Autodesk Inventor part; units mm, degrees
(part 4 of 5)
sketch "Sketch12" plane through (0, 0, 3) normal (0, 0, 1) x (1, 0, 0)
  line L0 (-25.3933, -129) -> (-25.3933, -146.5) projected
  line L1 (-25.3933, -146.5) -> (23.6067, -146.5) projected
  line L2 (23.6067, -146.5) -> (23.6067, -129) projected
  line L3 (23.6067, -129) -> (98, -129) projected
  line L4 (98, -129) -> (98, 184.5) projected
  line L5 (98, 184.5) -> (80.4, 184.5) projected
  line L6 (80.4, 184.5) -> (80.4, 215) projected
  line L7 (80.4, 215) -> (-78, 215) projected
  line L8 (-78, 215) -> (-78, 46.0635) projected
  line L9 (-78, 46.0635) -> (-75, 46.0635) projected
  line L10 (-75, 46.0635) -> (-75, 40.8932) projected
  line L11 (-75, 40.8932) -> (-78, 40.8932) projected
  line L12 (-78, 40.8932) -> (-78, 30.6062) projected
  line L13 (-78, 30.6062) -> (-75, 30.6062) projected
  line L14 (-75, 30.6062) -> (-75, 20.5478) projected
  line L15 (-75, 20.5478) -> (-78, 20.5478) projected
  line L16 (-78, 20.5478) -> (-78, 10.2608) projected
  line L17 (-78, 10.2608) -> (-75, 10.2608) projected
  line L18 (-75, 10.2608) -> (-75, -0.1068) projected
  line L19 (-75, -0.1068) -> (-78, -0.1068) projected
  line L20 (-78, -0.1068) -> (-78, -10.3938) projected
  line L21 (-78, -10.3938) -> (-75, -10.3938) projected
  line L22 (-75, -10.3938) -> (-75, -20.4522) projected
  line L23 (-75, -20.4522) -> (-78, -20.4522) projected
  line L24 (-78, -20.4522) -> (-78, -30.7392) projected
  line L25 (-78, -30.7392) -> (-75, -30.7392) projected
  line L26 (-75, -30.7392) -> (-75, -41.1068) projected
  line L27 (-75, -41.1068) -> (-78, -41.1068) projected
  line L28 (-78, -41.1068) -> (-78, -51.3938) projected
  line L29 (-78, -51.3938) -> (-75, -51.3938) projected
  line L30 (-75, -51.3938) -> (-75, -61.4522) projected
  line L31 (-75, -61.4522) -> (-78, -61.4522) projected
  line L32 (-78, -61.4522) -> (-78, -71.7392) projected
  line L33 (-78, -71.7392) -> (-75, -71.7392) projected
  line L34 (-75, -71.7392) -> (-75, -82.1068) projected
  line L35 (-75, -82.1068) -> (-78, -82.1068) projected
  line L36 (-78, -82.1068) -> (-78, -92.3938) projected
  line L37 (-78, -92.3938) -> (-75, -92.3938) projected
  line L38 (-75, -92.3938) -> (-75, -102.4522) projected
  line L39 (-75, -102.4522) -> (-78, -102.4522) projected
  line L40 (-78, -102.4522) -> (-78, -112.7392) projected
  line L41 (-78, -112.7392) -> (-75, -112.7392) projected
  line L42 (-75, -112.7392) -> (-75, -129) projected
  line L43 (-75, -129) -> (-25.3933, -129) projected
  circle A0 centre (88, 174.5) radius 2.25 projected
  circle A1 centre (88, 131.8987) radius 2.25 projected
  circle A2 centre (88, 58.3987) radius 2.25 projected
  circle A3 centre (88, -117.6237) radius 2.25 projected
  circle A4 centre (-17.8933, -140) radius 2.25 projected
  circle A5 centre (16.1067, -140) radius 2.25 projected
  line L44 (-58.9404, 10.4643) -> (-58.9404, 20.3443) projected
  arc A6 (-55.9404, 23.3443) -> (-58.9404, 20.3443) centre (-55.9404, 20.3443) ccw projected
  line L45 (-55.9404, 23.3443) -> (31.7396, 23.3443) projected
  arc A7 (34.7396, 20.3443) -> (31.7396, 23.3443) centre (31.7396, 20.3443) ccw projected
  line L46 (34.7396, 20.3443) -> (34.7396, 10.4643) projected
  arc A8 (31.7396, 7.4643) -> (34.7396, 10.4643) centre (31.7396, 10.4643) ccw projected
  line L47 (31.7396, 7.4643) -> (-55.9404, 7.4643) projected
  arc A9 (-58.9404, 10.4643) -> (-55.9404, 7.4643) centre (-55.9404, 10.4643) ccw projected
  line L48 (-58.9404, 30.8097) -> (-58.9404, 40.6897) projected
  arc A10 (-55.9404, 43.6897) -> (-58.9404, 40.6897) centre (-55.9404, 40.6897) ccw projected
  line L49 (-55.9404, 43.6897) -> (31.7396, 43.6897) projected
  arc A11 (34.7396, 40.6897) -> (31.7396, 43.6897) centre (31.7396, 40.6897) ccw projected
  line L50 (34.7396, 40.6897) -> (34.7396, 30.8097) projected
  arc A12 (31.7396, 27.8097) -> (34.7396, 30.8097) centre (31.7396, 30.8097) ccw projected
  line L51 (31.7396, 27.8097) -> (-55.9404, 27.8097) projected
  arc A13 (-58.9404, 30.8097) -> (-55.9404, 27.8097) centre (-55.9404, 30.8097) ccw projected
  arc A14 (-55.9404, 2.9989) -> (-58.9404, -0.0011) centre (-55.9404, -0.0011) ccw projected
  line L52 (-55.9404, 2.9989) -> (31.7396, 2.9989) projected
  arc A15 (34.7396, -0.0011) -> (31.7396, 2.9989) centre (31.7396, -0.0011) ccw projected
  line L53 (34.7396, -0.0011) -> (34.7396, -9.8811) projected
  arc A16 (31.7396, -12.8811) -> (34.7396, -9.8811) centre (31.7396, -9.8811) ccw projected
  line L54 (31.7396, -12.8811) -> (-55.9404, -12.8811) projected
  arc A17 (-58.9404, -9.8811) -> (-55.9404, -12.8811) centre (-55.9404, -9.8811) ccw projected
  line L55 (-58.9404, -9.8811) -> (-58.9404, -0.0011) projected
  arc A18 (-55.9404, -37.6919) -> (-58.9404, -40.6919) centre (-55.9404, -40.6919) ccw projected
  line L56 (-55.9404, -37.6919) -> (31.7396, -37.6919) projected
  arc A19 (34.7396, -40.6919) -> (31.7396, -37.6919) centre (31.7396, -40.6919) ccw projected
  line L57 (34.7396, -40.6919) -> (34.7396, -50.5719) projected
  arc A20 (31.7396, -53.5719) -> (34.7396, -50.5719) centre (31.7396, -50.5719) ccw projected
  line L58 (31.7396, -53.5719) -> (-55.9404, -53.5719) projected
  arc A21 (-58.9404, -50.5719) -> (-55.9404, -53.5719) centre (-55.9404, -50.5719) ccw projected
  line L59 (-58.9404, -50.5719) -> (-58.9404, -40.6919) projected
  line L60 (-55.9404, -58.0373) -> (31.7396, -58.0373) projected
  arc A22 (34.7396, -61.0373) -> (31.7396, -58.0373) centre (31.7396, -61.0373) ccw projected
  line L61 (34.7396, -61.0373) -> (34.7396, -70.9173) projected
  arc A23 (31.7396, -73.9173) -> (34.7396, -70.9173) centre (31.7396, -70.9173) ccw projected
  line L62 (31.7396, -73.9173) -> (-55.9404, -73.9173) projected
  arc A24 (-58.9404, -70.9173) -> (-55.9404, -73.9173) centre (-55.9404, -70.9173) ccw projected
  line L63 (-58.9404, -70.9173) -> (-58.9404, -61.0373) projected
  arc A25 (-55.9404, -58.0373) -> (-58.9404, -61.0373) centre (-55.9404, -61.0373) ccw projected
  line L64 (31.7396, -33.2265) -> (-55.9404, -33.2265) projected
  arc A26 (-58.9404, -30.2265) -> (-55.9404, -33.2265) centre (-55.9404, -30.2265) ccw projected
  line L65 (-58.9404, -30.2265) -> (-58.9404, -20.3465) projected
  arc A27 (-55.9404, -17.3465) -> (-58.9404, -20.3465) centre (-55.9404, -20.3465) ccw projected
  line L66 (-55.9404, -17.3465) -> (31.7396, -17.3465) projected
  arc A28 (34.7396, -20.3465) -> (31.7396, -17.3465) centre (31.7396, -20.3465) ccw projected
  line L67 (34.7396, -20.3465) -> (34.7396, -30.2265) projected
  arc A29 (31.7396, -33.2265) -> (34.7396, -30.2265) centre (31.7396, -30.2265) ccw projected
  arc A30 (34.7396, -81.3827) -> (31.7396, -78.3827) centre (31.7396, -81.3827) ccw projected
  line L68 (34.7396, -81.3827) -> (34.7396, -91.2627) projected
  arc A31 (31.7396, -94.2627) -> (34.7396, -91.2627) centre (31.7396, -91.2627) ccw projected
  line L69 (31.7396, -94.2627) -> (-55.9404, -94.2627) projected
  arc A32 (-58.9404, -91.2627) -> (-55.9404, -94.2627) centre (-55.9404, -91.2627) ccw projected
  line L70 (-58.9404, -91.2627) -> (-58.9404, -81.3827) projected
  arc A33 (-55.9404, -78.3827) -> (-58.9404, -81.3827) centre (-55.9404, -81.3827) ccw projected
  line L71 (-55.9404, -78.3827) -> (31.7396, -78.3827) projected
  arc A34 (31.7396, -114.6081) -> (34.7396, -111.6081) centre (31.7396, -111.6081) ccw projected
  line L72 (31.7396, -114.6081) -> (-55.9404, -114.6081) projected
  arc A35 (-58.9404, -111.6081) -> (-55.9404, -114.6081) centre (-55.9404, -111.6081) ccw projected
  line L73 (-58.9404, -111.6081) -> (-58.9404, -101.7281) projected
  arc A36 (-55.9404, -98.7281) -> (-58.9404, -101.7281) centre (-55.9404, -101.7281) ccw projected
  line L74 (-55.9404, -98.7281) -> (31.7396, -98.7281) projected
  arc A37 (34.7396, -101.7281) -> (31.7396, -98.7281) centre (31.7396, -101.7281) ccw projected
  line L75 (34.7396, -101.7281) -> (34.7396, -111.6081) projected
  line L76 (-69.3194, 50.0635) -> (-69.3194, 207.0635) projected
  arc A38 (-68.3194, 208.0635) -> (-69.3194, 207.0635) centre (-68.3194, 207.0635) ccw projected
  line L77 (-68.3194, 208.0635) -> (-25.6194, 208.0635) projected
  arc A39 (-24.6194, 207.0635) -> (-25.6194, 208.0635) centre (-25.6194, 207.0635) ccw projected
  line L78 (-24.6194, 207.0635) -> (-24.6194, 50.0635) projected
  arc A40 (-25.6194, 49.0635) -> (-24.6194, 50.0635) centre (-25.6194, 50.0635) ccw projected
  line L79 (-25.6194, 49.0635) -> (-68.3194, 49.0635) projected
  arc A41 (-69.3194, 50.0635) -> (-68.3194, 49.0635) centre (-68.3194, 50.0635) ccw projected
  line L80 (64, 48.3987) -> (64, -109.7094) projected
  arc A42 (63.7071, -110.4166) -> (64, -109.7094) centre (63, -109.7094) ccw projected
  line L81 (63.7071, -110.4166) -> (59.2929, -114.8308) projected
  arc A43 (58.5858, -115.1237) -> (59.2929, -114.8308) centre (58.5858, -114.1237) ccw projected
  line L82 (58.5858, -115.1237) -> (43.2196, -115.1237) projected
  arc A44 (42.2196, -114.1237) -> (43.2196, -115.1237) centre (43.2196, -114.1237) ccw projected
  line L83 (42.2196, -114.1237) -> (42.2196, -104.6674) projected
  arc A45 (42.2196, -104.6674) -> (40.773, -102.7455) centre (40.2196, -104.6674) ccw projected
  arc A46 (39.7673, -102.1811) -> (40.773, -102.7455) centre (41.4696, -100.3262) ccw projected
  arc A47 (39.1196, -100.7076) -> (39.7673, -102.1811) centre (41.1196, -100.7076) ccw projected
  line L84 (39.1196, -100.7076) -> (39.1196, -95.7515) projected
  arc A48 (39.7673, -94.2779) -> (39.1196, -95.7515) centre (41.1196, -95.7515) ccw projected
  arc A49 (39.937, -94.1354) -> (39.7673, -94.2779) centre (41.4696, -96.1328) ccw projected
  arc A50 (39.937, -94.1354) -> (40.7196, -92.5486) centre (38.7196, -92.5486) ccw projected
  line L85 (40.7196, -92.5486) -> (40.7196, -83.4104) projected
  arc A51 (40.7196, -83.4104) -> (39.937, -81.8236) centre (38.7196, -83.4104) ccw projected
  arc A52 (39.7673, -81.6811) -> (39.937, -81.8236) centre (41.4696, -79.8262) ccw projected
  arc A53 (39.1196, -80.2076) -> (39.7673, -81.6811) centre (41.1196, -80.2076) ccw projected
  line L86 (39.1196, -80.2076) -> (39.1196, -75.2515) projected
  arc A54 (39.7673, -73.7779) -> (39.1196, -75.2515) centre (41.1196, -75.2515) ccw projected
  arc A55 (39.937, -73.6354) -> (39.7673, -73.7779) centre (41.4696, -75.6328) ccw projected
  arc A56 (39.937, -73.6354) -> (40.7196, -72.0486) centre (38.7196, -72.0486) ccw projected
  line L87 (40.7196, -72.0486) -> (40.7196, -62.9104) projected
  arc A57 (40.7196, -62.9104) -> (39.937, -61.3236) centre (38.7196, -62.9104) ccw projected
  arc A58 (39.7673, -61.1811) -> (39.937, -61.3236) centre (41.4696, -59.3262) ccw projected
  arc A59 (39.1196, -59.7076) -> (39.7673, -61.1811) centre (41.1196, -59.7076) ccw projected
  line L88 (39.1196, -59.7076) -> (39.1196, -54.7515) projected
  arc A60 (39.7673, -53.2779) -> (39.1196, -54.7515) centre (41.1196, -54.7515) ccw projected
  arc A61 (39.937, -53.1354) -> (39.7673, -53.2779) centre (41.4696, -55.1328) ccw projected
  arc A62 (39.937, -53.1354) -> (40.7196, -51.5486) centre (38.7196, -51.5486) ccw projected
  line L89 (40.7196, -51.5486) -> (40.7196, -42.4104) projected
  arc A63 (40.7196, -42.4104) -> (39.937, -40.8236) centre (38.7196, -42.4104) ccw projected
  arc A64 (39.7673, -40.6811) -> (39.937, -40.8236) centre (41.4696, -38.8262) ccw projected
  arc A65 (39.1196, -39.2076) -> (39.7673, -40.6811) centre (41.1196, -39.2076) ccw projected
  line L90 (39.1196, -39.2076) -> (39.1196, -34.2515) projected
  arc A66 (39.7673, -32.7779) -> (39.1196, -34.2515) centre (41.1196, -34.2515) ccw projected
  arc A67 (39.937, -32.6354) -> (39.7673, -32.7779) centre (41.4696, -34.6328) ccw projected
  arc A68 (39.937, -32.6354) -> (40.7196, -31.0486) centre (38.7196, -31.0486) ccw projected
  line L91 (40.7196, -31.0486) -> (40.7196, -21.9104) projected
  arc A69 (40.7196, -21.9104) -> (39.937, -20.3236) centre (38.7196, -21.9104) ccw projected
  arc A70 (39.7673, -20.1811) -> (39.937, -20.3236) centre (41.4696, -18.3262) ccw projected
  arc A71 (39.1196, -18.7076) -> (39.7673, -20.1811) centre (41.1196, -18.7076) ccw projected
  line L92 (39.1196, -18.7076) -> (39.1196, -13.7515) projected
  arc A72 (39.7673, -12.2779) -> (39.1196, -13.7515) centre (41.1196, -13.7515) ccw projected
  arc A73 (39.937, -12.1354) -> (39.7673, -12.2779) centre (41.4696, -14.1328) ccw projected
  arc A74 (39.937, -12.1354) -> (40.7196, -10.5486) centre (38.7196, -10.5486) ccw projected
  line L93 (40.7196, -10.5486) -> (40.7196, -1.4104) projected
  arc A75 (40.7196, -1.4104) -> (39.937, 0.1764) centre (38.7196, -1.4104) ccw projected
  arc A76 (39.7673, 0.3189) -> (39.937, 0.1764) centre (41.4696, 2.1738) ccw projected
  arc A77 (39.1196, 1.7924) -> (39.7673, 0.3189) centre (41.1196, 1.7924) ccw projected
  line L94 (39.1196, 1.7924) -> (39.1196, 6.7485) projected
  arc A78 (39.7673, 8.2221) -> (39.1196, 6.7485) centre (41.1196, 6.7485) ccw projected
  arc A79 (39.937, 8.3646) -> (39.7673, 8.2221) centre (41.4696, 6.3672) ccw projected
  arc A80 (39.937, 8.3646) -> (40.7196, 9.9514) centre (38.7196, 9.9514) ccw projected
  line L95 (40.7196, 9.9514) -> (40.7196, 19.0896) projected
  arc A81 (40.7196, 19.0896) -> (39.937, 20.6764) centre (38.7196, 19.0896) ccw projected
  arc A82 (39.7673, 20.8189) -> (39.937, 20.6764) centre (41.4696, 22.6738) ccw projected
  arc A83 (39.1196, 22.2924) -> (39.7673, 20.8189) centre (41.1196, 22.2924) ccw projected
  line L96 (39.1196, 22.2924) -> (39.1196, 27.2485) projected
  arc A84 (39.7673, 28.7221) -> (39.1196, 27.2485) centre (41.1196, 27.2485) ccw projected
  arc A85 (39.937, 28.8646) -> (39.7673, 28.7221) centre (41.4696, 26.8672) ccw projected
  arc A86 (39.937, 28.8646) -> (40.7196, 30.4514) centre (38.7196, 30.4514) ccw projected
  line L97 (40.7196, 30.4514) -> (40.7196, 39.5896) projected
  arc A87 (40.7196, 39.5896) -> (39.937, 41.1764) centre (38.7196, 39.5896) ccw projected
  arc A88 (39.7673, 41.3189) -> (39.937, 41.1764) centre (41.4696, 43.1738) ccw projected
  arc A89 (39.1196, 42.7924) -> (39.7673, 41.3189) centre (41.1196, 42.7924) ccw projected
  line L98 (39.1196, 42.7924) -> (39.1196, 47.7485) projected
  arc A90 (39.7673, 49.2221) -> (39.1196, 47.7485) centre (41.1196, 47.7485) ccw projected
  arc A91 (43.3362, 49.0566) -> (39.7673, 49.2221) centre (41.4696, 47.3672) ccw projected
  arc A92 (43.3362, 49.0566) -> (44.819, 48.3987) centre (44.819, 50.3987) ccw projected
  line L99 (44.819, 48.3987) -> (64, 48.3987) projected
  line L100 (17.2903, 185.473) -> (38.4903, 185.473)
  line L101 (41.4903, 188.473) -> (41.4903, 201.673)
  line L102 (38.4903, 204.673) -> (17.2903, 204.673)
  line L103 (14.2903, 201.673) -> (14.2903, 188.473)
  arc A93 (38.4903, 185.473) -> (41.4903, 188.473) centre (38.4903, 188.473) ccw
  arc A94 (41.4903, 201.673) -> (38.4903, 204.673) centre (38.4903, 201.673) ccw
  arc A95 (17.2903, 204.673) -> (14.2903, 201.673) centre (17.2903, 201.673) ccw
  arc A96 (14.2903, 188.473) -> (17.2903, 185.473) centre (17.2903, 188.473) ccw
  circle A97 centre (47.8903, 195.073) radius 1.75
  circle A98 centre (7.8903, 195.073) radius 1.75
  line L104 (15.5287, 72.6659) -> (40.2515, 72.6659)
  line L105 (40.2515, 150.2659) -> (15.5287, 150.2659)
  line L106 (-8.1099, 127.2849) -> (-8.1099, 95.6469)
  arc A99 (-8.1099, 95.6469) -> (-2.1613, 81.4146) centre (11.8901, 95.6469) ccw
  arc A100 (4.5403, 75.9549) -> (15.5287, 72.6659) centre (15.5287, 92.6659) ccw
  arc A101 (-2.1615, 81.4137) -> (4.5403, 75.9549) centre (27.8907, 111.4659) ccw
  line L107 (27.8901, 106.1082) -> (27.8901, 119.1725)
  line L108 (22.3518, 111.4659) -> (33.8609, 111.4659)
  arc A102 (-2.1613, 141.5172) -> (-8.1099, 127.2849) centre (11.8901, 127.2849) ccw
  arc A103 (15.5287, 150.2659) -> (4.5403, 146.9769) centre (15.5287, 130.2659) ccw
  arc A104 (4.5403, 146.9769) -> (-2.1615, 141.5181) centre (27.8907, 111.4659) ccw
  line L109 (63.8901, 95.6469) -> (63.8901, 127.2849)
  arc A105 (4.5403, 146.9769) -> (-2.1615, 141.5181) centre (27.8907, 111.4659) ccw
  circle A106 centre (-7.8093, 75.7659) radius 1.2
  circle A107 centre (63.5895, 75.7659) radius 1.2
  circle A108 centre (-7.8093, 147.1659) radius 1.2
  circle A109 centre (63.5895, 147.1659) radius 1.2
  circle A110 centre (88, -117.6237) radius 2.25 projected
  circle A111 centre (88, 58.3987) radius 2.25 projected
  circle A112 centre (88, 131.8987) radius 2.25 projected
  circle A113 centre (88, 174.5) radius 2.25 projected
  line L110 (64, -109.7094) -> (64, 48.3987) projected
  line L111 (64, 48.3987) -> (44.819, 48.3987) projected
  arc A114 (43.3362, 49.0566) -> (44.819, 48.3987) centre (44.819, 50.3987) ccw projected
  arc A115 (43.3362, 49.0566) -> (39.7673, 49.2221) centre (41.4696, 47.3672) ccw projected
  arc A116 (39.7673, 49.2221) -> (39.1196, 47.7485) centre (41.1196, 47.7485) ccw projected
  line L112 (39.1196, 47.7485) -> (39.1196, 42.7924) projected
  arc A117 (39.1196, 42.7924) -> (39.7673, 41.3189) centre (41.1196, 42.7924) ccw projected
  arc A118 (39.7673, 41.3189) -> (39.937, 41.1764) centre (41.4696, 43.1738) ccw projected
  arc A119 (40.7196, 39.5896) -> (39.937, 41.1764) centre (38.7196, 39.5896) ccw projected
  line L113 (40.7196, 39.5896) -> (40.7196, 30.4514) projected
  arc A120 (39.937, 28.8646) -> (40.7196, 30.4514) centre (38.7196, 30.4514) ccw projected
  arc A121 (39.937, 28.8646) -> (39.7673, 28.7221) centre (41.4696, 26.8672) ccw projected
  arc A122 (39.7673, 28.7221) -> (39.1196, 27.2485) centre (41.1196, 27.2485) ccw projected
  line L114 (39.1196, 27.2485) -> (39.1196, 22.2924) projected
  arc A123 (39.1196, 22.2924) -> (39.7673, 20.8189) centre (41.1196, 22.2924) ccw projected
  arc A124 (39.7673, 20.8189) -> (39.937, 20.6764) centre (41.4696, 22.6738) ccw projected
  arc A125 (40.7196, 19.0896) -> (39.937, 20.6764) centre (38.7196, 19.0896) ccw projected
  line L115 (40.7196, 19.0896) -> (40.7196, 9.9514) projected
  arc A126 (39.937, 8.3646) -> (40.7196, 9.9514) centre (38.7196, 9.9514) ccw projected
  arc A127 (39.937, 8.3646) -> (39.7673, 8.2221) centre (41.4696, 6.3672) ccw projected
  arc A128 (39.7673, 8.2221) -> (39.1196, 6.7485) centre (41.1196, 6.7485) ccw projected
  line L116 (39.1196, 6.7485) -> (39.1196, 1.7924) projected
  arc A129 (39.1196, 1.7924) -> (39.7673, 0.3189) centre (41.1196, 1.7924) ccw projected
  arc A130 (39.7673, 0.3189) -> (39.937, 0.1764) centre (41.4696, 2.1738) ccw projected
  arc A131 (40.7196, -1.4104) -> (39.937, 0.1764) centre (38.7196, -1.4104) ccw projected
  line L117 (40.7196, -1.4104) -> (40.7196, -10.5486) projected
  arc A132 (39.937, -12.1354) -> (40.7196, -10.5486) centre (38.7196, -10.5486) ccw projected
  arc A133 (39.937, -12.1354) -> (39.7673, -12.2779) centre (41.4696, -14.1328) ccw projected
  arc A134 (39.7673, -12.2779) -> (39.1196, -13.7515) centre (41.1196, -13.7515) ccw projected
  line L118 (39.1196, -13.7515) -> (39.1196, -18.7076) projected
  arc A135 (39.1196, -18.7076) -> (39.7673, -20.1811) centre (41.1196, -18.7076) ccw projected
  arc A136 (39.7673, -20.1811) -> (39.937, -20.3236) centre (41.4696, -18.3262) ccw projected
  arc A137 (40.7196, -21.9104) -> (39.937, -20.3236) centre (38.7196, -21.9104) ccw projected
  line L119 (40.7196, -21.9104) -> (40.7196, -31.0486) projected
  arc A138 (39.937, -32.6354) -> (40.7196, -31.0486) centre (38.7196, -31.0486) ccw projected
  arc A139 (39.937, -32.6354) -> (39.7673, -32.7779) centre (41.4696, -34.6328) ccw projected
  arc A140 (39.7673, -32.7779) -> (39.1196, -34.2515) centre (41.1196, -34.2515) ccw projected
  line L120 (39.1196, -34.2515) -> (39.1196, -39.2076) projected
  arc A141 (39.1196, -39.2076) -> (39.7673, -40.6811) centre (41.1196, -39.2076) ccw projected
  arc A142 (39.7673, -40.6811) -> (39.937, -40.8236) centre (41.4696, -38.8262) ccw projected
  arc A143 (40.7196, -42.4104) -> (39.937, -40.8236) centre (38.7196, -42.4104) ccw projected
  line L121 (40.7196, -42.4104) -> (40.7196, -51.5486) projected
  arc A144 (39.937, -53.1354) -> (40.7196, -51.5486) centre (38.7196, -51.5486) ccw projected
  arc A145 (39.937, -53.1354) -> (39.7673, -53.2779) centre (41.4696, -55.1328) ccw projected
  arc A146 (39.7673, -53.2779) -> (39.1196, -54.7515) centre (41.1196, -54.7515) ccw projected
  line L122 (39.1196, -54.7515) -> (39.1196, -59.7076) projected
  arc A147 (39.1196, -59.7076) -> (39.7673, -61.1811) centre (41.1196, -59.7076) ccw projected
  arc A148 (39.7673, -61.1811) -> (39.937, -61.3236) centre (41.4696, -59.3262) ccw projected
  arc A149 (40.7196, -62.9104) -> (39.937, -61.3236) centre (38.7196, -62.9104) ccw projected
  line L123 (40.7196, -62.9104) -> (40.7196, -72.0486) projected
  arc A150 (39.937, -73.6354) -> (40.7196, -72.0486) centre (38.7196, -72.0486) ccw projected
  arc A151 (39.937, -73.6354) -> (39.7673, -73.7779) centre (41.4696, -75.6328) ccw projected
  arc A152 (39.7673, -73.7779) -> (39.1196, -75.2515) centre (41.1196, -75.2515) ccw projected
  line L124 (39.1196, -75.2515) -> (39.1196, -80.2076) projected
  arc A153 (39.1196, -80.2076) -> (39.7673, -81.6811) centre (41.1196, -80.2076) ccw projected
  arc A154 (39.7673, -81.6811) -> (39.937, -81.8236) centre (41.4696, -79.8262) ccw projected
  arc A155 (40.7196, -83.4104) -> (39.937, -81.8236) centre (38.7196, -83.4104) ccw projected
  line L125 (40.7196, -83.4104) -> (40.7196, -92.5486) projected
  arc A156 (39.937, -94.1354) -> (40.7196, -92.5486) centre (38.7196, -92.5486) ccw projected
  arc A157 (39.937, -94.1354) -> (39.7673, -94.2779) centre (41.4696, -96.1328) ccw projected
  arc A158 (39.7673, -94.2779) -> (39.1196, -95.7515) centre (41.1196, -95.7515) ccw projected
  line L126 (39.1196, -95.7515) -> (39.1196, -100.7076) projected
  arc A159 (39.1196, -100.7076) -> (39.7673, -102.1811) centre (41.1196, -100.7076) ccw projected
  arc A160 (39.7673, -102.1811) -> (40.773, -102.7455) centre (41.4696, -100.3262) ccw projected
  arc A161 (42.2196, -104.6674) -> (40.773, -102.7455) centre (40.2196, -104.6674) ccw projected
  line L127 (42.2196, -104.6674) -> (42.2196, -114.1237) projected
  arc A162 (42.2196, -114.1237) -> (43.2196, -115.1237) centre (43.2196, -114.1237) ccw projected
  line L128 (43.2196, -115.1237) -> (58.5858, -115.1237) projected
  arc A163 (58.5858, -115.1237) -> (59.2929, -114.8308) centre (58.5858, -114.1237) ccw projected
  line L129 (59.2929, -114.8308) -> (63.7071, -110.4166) projected
  arc A164 (63.7071, -110.4166) -> (64, -109.7094) centre (63, -109.7094) ccw projected
  line L130 (-69.3194, 207.0635) -> (-69.3194, 50.0635) projected
  arc A165 (-69.3194, 50.0635) -> (-68.3194, 49.0635) centre (-68.3194, 50.0635) ccw projected
  line L131 (-68.3194, 49.0635) -> (-25.6194, 49.0635) projected
  arc A166 (-25.6194, 49.0635) -> (-24.6194, 50.0635) centre (-25.6194, 50.0635) ccw projected
  line L132 (-24.6194, 50.0635) -> (-24.6194, 207.0635) projected
  arc A167 (-24.6194, 207.0635) -> (-25.6194, 208.0635) centre (-25.6194, 207.0635) ccw projected
  line L133 (-25.6194, 208.0635) -> (-68.3194, 208.0635) projected
  arc A168 (-68.3194, 208.0635) -> (-69.3194, 207.0635) centre (-68.3194, 207.0635) ccw projected
  arc A169 (31.7396, -114.6081) -> (34.7396, -111.6081) centre (31.7396, -111.6081) ccw projected
  line L134 (34.7396, -111.6081) -> (34.7396, -101.7281) projected
  arc A170 (34.7396, -101.7281) -> (31.7396, -98.7281) centre (31.7396, -101.7281) ccw projected
  line L135 (31.7396, -98.7281) -> (-55.9404, -98.7281) projected
  arc A171 (-55.9404, -98.7281) -> (-58.9404, -101.7281) centre (-55.9404, -101.7281) ccw projected
  line L136 (-58.9404, -101.7281) -> (-58.9404, -111.6081) projected
  arc A172 (-58.9404, -111.6081) -> (-55.9404, -114.6081) centre (-55.9404, -111.6081) ccw projected
  line L137 (-55.9404, -114.6081) -> (31.7396, -114.6081) projected
  arc A173 (34.7396, -81.3827) -> (31.7396, -78.3827) centre (31.7396, -81.3827) ccw projected
  line L138 (31.7396, -78.3827) -> (-55.9404, -78.3827) projected
  arc A174 (-55.9404, -78.3827) -> (-58.9404, -81.3827) centre (-55.9404, -81.3827) ccw projected
  line L139 (-58.9404, -81.3827) -> (-58.9404, -91.2627) projected
  arc A175 (-58.9404, -91.2627) -> (-55.9404, -94.2627) centre (-55.9404, -91.2627) ccw projected
  line L140 (-55.9404, -94.2627) -> (31.7396, -94.2627) projected
  arc A176 (31.7396, -94.2627) -> (34.7396, -91.2627) centre (31.7396, -91.2627) ccw projected
  line L141 (34.7396, -91.2627) -> (34.7396, -81.3827) projected
  line L142 (-55.9404, -33.2265) -> (31.7396, -33.2265) projected
  arc A177 (31.7396, -33.2265) -> (34.7396, -30.2265) centre (31.7396, -30.2265) ccw projected
  line L143 (34.7396, -30.2265) -> (34.7396, -20.3465) projected
  arc A178 (34.7396, -20.3465) -> (31.7396, -17.3465) centre (31.7396, -20.3465) ccw projected
  line L144 (31.7396, -17.3465) -> (-55.9404, -17.3465) projected
  arc A179 (-55.9404, -17.3465) -> (-58.9404, -20.3465) centre (-55.9404, -20.3465) ccw projected
  line L145 (-58.9404, -20.3465) -> (-58.9404, -30.2265) projected
  arc A180 (-58.9404, -30.2265) -> (-55.9404, -33.2265) centre (-55.9404, -30.2265) ccw projected
  line L146 (31.7396, -58.0373) -> (-55.9404, -58.0373) projected
  arc A181 (-55.9404, -58.0373) -> (-58.9404, -61.0373) centre (-55.9404, -61.0373) ccw projected
  line L147 (-58.9404, -61.0373) -> (-58.9404, -70.9173) projected
  arc A182 (-58.9404, -70.9173) -> (-55.9404, -73.9173) centre (-55.9404, -70.9173) ccw projected
  line L148 (-55.9404, -73.9173) -> (31.7396, -73.9173) projected
  arc A183 (31.7396, -73.9173) -> (34.7396, -70.9173) centre (31.7396, -70.9173) ccw projected
  line L149 (34.7396, -70.9173) -> (34.7396, -61.0373) projected
  arc A184 (34.7396, -61.0373) -> (31.7396, -58.0373) centre (31.7396, -61.0373) ccw projected
  arc A185 (-55.9404, -37.6919) -> (-58.9404, -40.6919) centre (-55.9404, -40.6919) ccw projected
  line L150 (-58.9404, -40.6919) -> (-58.9404, -50.5719) projected
  arc A186 (-58.9404, -50.5719) -> (-55.9404, -53.5719) centre (-55.9404, -50.5719) ccw projected
  line L151 (-55.9404, -53.5719) -> (31.7396, -53.5719) projected
  arc A187 (31.7396, -53.5719) -> (34.7396, -50.5719) centre (31.7396, -50.5719) ccw projected
  line L152 (34.7396, -50.5719) -> (34.7396, -40.6919) projected
  arc A188 (34.7396, -40.6919) -> (31.7396, -37.6919) centre (31.7396, -40.6919) ccw projected
  line L153 (31.7396, -37.6919) -> (-55.9404, -37.6919) projected
  arc A189 (-55.9404, 2.9989) -> (-58.9404, -0.0011) centre (-55.9404, -0.0011) ccw projected
  line L154 (-58.9404, -0.0011) -> (-58.9404, -9.8811) projected
  arc A190 (-58.9404, -9.8811) -> (-55.9404, -12.8811) centre (-55.9404, -9.8811) ccw projected
  line L155 (-55.9404, -12.8811) -> (31.7396, -12.8811) projected
  arc A191 (31.7396, -12.8811) -> (34.7396, -9.8811) centre (31.7396, -9.8811) ccw projected
  line L156 (34.7396, -9.8811) -> (34.7396, -0.0011) projected
  arc A192 (34.7396, -0.0011) -> (31.7396, 2.9989) centre (31.7396, -0.0011) ccw projected
  line L157 (31.7396, 2.9989) -> (-55.9404, 2.9989) projected
  line L158 (-58.9404, 40.6897) -> (-58.9404, 30.8097) projected
  arc A193 (-58.9404, 30.8097) -> (-55.9404, 27.8097) centre (-55.9404, 30.8097) ccw projected
  line L159 (-55.9404, 27.8097) -> (31.7396, 27.8097) projected
  arc A194 (31.7396, 27.8097) -> (34.7396, 30.8097) centre (31.7396, 30.8097) ccw projected
  line L160 (34.7396, 30.8097) -> (34.7396, 40.6897) projected
  arc A195 (34.7396, 40.6897) -> (31.7396, 43.6897) centre (31.7396, 40.6897) ccw projected
  line L161 (31.7396, 43.6897) -> (-55.9404, 43.6897) projected
  arc A196 (-55.9404, 43.6897) -> (-58.9404, 40.6897) centre (-55.9404, 40.6897) ccw projected
  line L162 (-58.9404, 20.3443) -> (-58.9404, 10.4643) projected
  arc A197 (-58.9404, 10.4643) -> (-55.9404, 7.4643) centre (-55.9404, 10.4643) ccw projected
  line L163 (-55.9404, 7.4643) -> (31.7396, 7.4643) projected
  arc A198 (31.7396, 7.4643) -> (34.7396, 10.4643) centre (31.7396, 10.4643) ccw projected
  line L164 (34.7396, 10.4643) -> (34.7396, 20.3443) projected
  arc A199 (34.7396, 20.3443) -> (31.7396, 23.3443) centre (31.7396, 20.3443) ccw projected
  line L165 (31.7396, 23.3443) -> (-55.9404, 23.3443) projected
  arc A200 (-55.9404, 23.3443) -> (-58.9404, 20.3443) centre (-55.9404, 20.3443) ccw projected
  circle A201 centre (16.1067, -140) radius 2.25 projected
  circle A202 centre (-17.8933, -140) radius 2.25 projected
  line L166 (-75, 46.0635) -> (-78, 46.0635) projected
  line L167 (-78, 46.0635) -> (-78, 215) projected
  line L168 (-78, 215) -> (80.4, 215) projected
  line L169 (80.4, 215) -> (80.4, 184.5) projected
  line L170 (80.4, 184.5) -> (98, 184.5) projected
  line L171 (98, 184.5) -> (98, -129) projected
  line L172 (98, -129) -> (23.6067, -129) projected
  line L173 (23.6067, -129) -> (23.6067, -146.5) projected
  line L174 (23.6067, -146.5) -> (-25.3933, -146.5) projected
  line L175 (-25.3933, -146.5) -> (-25.3933, -129) projected
  line L176 (-25.3933, -129) -> (-75, -129) projected
  line L177 (-75, -129) -> (-75, -112.7392) projected
  line L178 (-75, -112.7392) -> (-78, -112.7392) projected
  line L179 (-78, -112.7392) -> (-78, -102.4522) projected
  line L180 (-78, -102.4522) -> (-75, -102.4522) projected
  line L181 (-75, -102.4522) -> (-75, -92.3938) projected
  line L182 (-75, -92.3938) -> (-78, -92.3938) projected
  line L183 (-78, -92.3938) -> (-78, -82.1068) projected
  line L184 (-78, -82.1068) -> (-75, -82.1068) projected
  line L185 (-75, -82.1068) -> (-75, -71.7392) projected
  line L186 (-75, -71.7392) -> (-78, -71.7392) projected
  line L187 (-78, -71.7392) -> (-78, -61.4522) projected
  line L188 (-78, -61.4522) -> (-75, -61.4522) projected
  line L189 (-75, -61.4522) -> (-75, -51.3938) projected
  line L190 (-75, -51.3938) -> (-78, -51.3938) projected
  line L191 (-78, -51.3938) -> (-78, -41.1068) projected
  line L192 (-78, -41.1068) -> (-75, -41.1068) projected
  line L193 (-75, -41.1068) -> (-75, -30.7392) projected
  line L194 (-75, -30.7392) -> (-78, -30.7392) projected
  line L195 (-78, -30.7392) -> (-78, -20.4522) projected
  line L196 (-78, -20.4522) -> (-75, -20.4522) projected
  line L197 (-75, -20.4522) -> (-75, -10.3938) projected
  line L198 (-75, -10.3938) -> (-78, -10.3938) projected
  line L199 (-78, -10.3938) -> (-78, -0.1068) projected
  line L200 (-78, -0.1068) -> (-75, -0.1068) projected
  line L201 (-75, -0.1068) -> (-75, 10.2608) projected
  line L202 (-75, 10.2608) -> (-78, 10.2608) projected
  line L203 (-78, 10.2608) -> (-78, 20.5478) projected
  line L204 (-78, 20.5478) -> (-75, 20.5478) projected
  line L205 (-75, 20.5478) -> (-75, 30.6062) projected
  line L206 (-75, 30.6062) -> (-78, 30.6062) projected
  line L207 (-78, 30.6062) -> (-78, 40.8932) projected
  line L208 (-78, 40.8932) -> (-75, 40.8932) projected
  line L209 (-75, 40.8932) -> (-75, 46.0635) projected
  circle A203 centre (88, -117.6237) radius 2.25 projected
  circle A204 centre (88, 58.3987) radius 2.25 projected
  circle A205 centre (88, 131.8987) radius 2.25 projected
  circle A206 centre (88, 174.5) radius 2.25 projected
  line L210 (64, -109.7094) -> (64, 48.3987) projected
  line L211 (64, 48.3987) -> (44.819, 48.3987) projected
  arc A207 (43.3362, 49.0566) -> (44.819, 48.3987) centre (44.819, 50.3987) ccw projected
  arc A208 (43.3362, 49.0566) -> (39.7673, 49.2221) centre (41.4696, 47.3672) ccw projected
  arc A209 (39.7673, 49.2221) -> (39.1196, 47.7485) centre (41.1196, 47.7485) ccw projected
  line L212 (39.1196, 47.7485) -> (39.1196, 42.7924) projected
  arc A210 (39.1196, 42.7924) -> (39.7673, 41.3189) centre (41.1196, 42.7924) ccw projected
  arc A211 (39.7673, 41.3189) -> (39.937, 41.1764) centre (41.4696, 43.1738) ccw projected
  arc A212 (40.7196, 39.5896) -> (39.937, 41.1764) centre (38.7196, 39.5896) ccw projected
  line L213 (40.7196, 39.5896) -> (40.7196, 30.4514) projected
  arc A213 (39.937, 28.8646) -> (40.7196, 30.4514) centre (38.7196, 30.4514) ccw projected
  arc A214 (39.937, 28.8646) -> (39.7673, 28.7221) centre (41.4696, 26.8672) ccw projected
  arc A215 (39.7673, 28.7221) -> (39.1196, 27.2485) centre (41.1196, 27.2485) ccw projected
  line L214 (39.1196, 27.2485) -> (39.1196, 22.2924) projected
  arc A216 (39.1196, 22.2924) -> (39.7673, 20.8189) centre (41.1196, 22.2924) ccw projected
  arc A217 (39.7673, 20.8189) -> (39.937, 20.6764) centre (41.4696, 22.6738) ccw projected
  arc A218 (40.7196, 19.0896) -> (39.937, 20.6764) centre (38.7196, 19.0896) ccw projected
  line L215 (40.7196, 19.0896) -> (40.7196, 9.9514) projected
  arc A219 (39.937, 8.3646) -> (40.7196, 9.9514) centre (38.7196, 9.9514) ccw projected
  arc A220 (39.937, 8.3646) -> (39.7673, 8.2221) centre (41.4696, 6.3672) ccw projected
  arc A221 (39.7673, 8.2221) -> (39.1196, 6.7485) centre (41.1196, 6.7485) ccw projected
  line L216 (39.1196, 6.7485) -> (39.1196, 1.7924) projected
  arc A222 (39.1196, 1.7924) -> (39.7673, 0.3189) centre (41.1196, 1.7924) ccw projected
  arc A223 (39.7673, 0.3189) -> (39.937, 0.1764) centre (41.4696, 2.1738) ccw projected
  arc A224 (40.7196, -1.4104) -> (39.937, 0.1764) centre (38.7196, -1.4104) ccw projected
  line L217 (40.7196, -1.4104) -> (40.7196, -10.5486) projected
  arc A225 (39.937, -12.1354) -> (40.7196, -10.5486) centre (38.7196, -10.5486) ccw projected
  arc A226 (39.937, -12.1354) -> (39.7673, -12.2779) centre (41.4696, -14.1328) ccw projected
  arc A227 (39.7673, -12.2779) -> (39.1196, -13.7515) centre (41.1196, -13.7515) ccw projected
  line L218 (39.1196, -13.7515) -> (39.1196, -18.7076) projected
  arc A228 (39.1196, -18.7076) -> (39.7673, -20.1811) centre (41.1196, -18.7076) ccw projected
  arc A229 (39.7673, -20.1811) -> (39.937, -20.3236) centre (41.4696, -18.3262) ccw projected
  arc A230 (40.7196, -21.9104) -> (39.937, -20.3236) centre (38.7196, -21.9104) ccw projected
  line L219 (40.7196, -21.9104) -> (40.7196, -31.0486) projected
  arc A231 (39.937, -32.6354) -> (40.7196, -31.0486) centre (38.7196, -31.0486) ccw projected
  arc A232 (39.937, -32.6354) -> (39.7673, -32.7779) centre (41.4696, -34.6328) ccw projected
  arc A233 (39.7673, -32.7779) -> (39.1196, -34.2515) centre (41.1196, -34.2515) ccw projected
  line L220 (39.1196, -34.2515) -> (39.1196, -39.2076) projected
  arc A234 (39.1196, -39.2076) -> (39.7673, -40.6811) centre (41.1196, -39.2076) ccw projected
  arc A235 (39.7673, -40.6811) -> (39.937, -40.8236) centre (41.4696, -38.8262) ccw projected
  arc A236 (40.7196, -42.4104) -> (39.937, -40.8236) centre (38.7196, -42.4104) ccw projected
  line L221 (40.7196, -42.4104) -> (40.7196, -51.5486) projected
  arc A237 (39.937, -53.1354) -> (40.7196, -51.5486) centre (38.7196, -51.5486) ccw projected
  arc A238 (39.937, -53.1354) -> (39.7673, -53.2779) centre (41.4696, -55.1328) ccw projected
  arc A239 (39.7673, -53.2779) -> (39.1196, -54.7515) centre (41.1196, -54.7515) ccw projected
  line L222 (39.1196, -54.7515) -> (39.1196, -59.7076) projected
  arc A240 (39.1196, -59.7076) -> (39.7673, -61.1811) centre (41.1196, -59.7076) ccw projected
  arc A241 (39.7673, -61.1811) -> (39.937, -61.3236) centre (41.4696, -59.3262) ccw projected
  arc A242 (40.7196, -62.9104) -> (39.937, -61.3236) centre (38.7196, -62.9104) ccw projected
  line L223 (40.7196, -62.9104) -> (40.7196, -72.0486) projected
  arc A243 (39.937, -73.6354) -> (40.7196, -72.0486) centre (38.7196, -72.0486) ccw projected
  arc A244 (39.937, -73.6354) -> (39.7673, -73.7779) centre (41.4696, -75.6328) ccw projected
  arc A245 (39.7673, -73.7779) -> (39.1196, -75.2515) centre (41.1196, -75.2515) ccw projected
  line L224 (39.1196, -75.2515) -> (39.1196, -80.2076) projected
  arc A246 (39.1196, -80.2076) -> (39.7673, -81.6811) centre (41.1196, -80.2076) ccw projected
  arc A247 (39.7673, -81.6811) -> (39.937, -81.8236) centre (41.4696, -79.8262) ccw projected
  arc A248 (40.7196, -83.4104) -> (39.937, -81.8236) centre (38.7196, -83.4104) ccw projected
  line L225 (40.7196, -83.4104) -> (40.7196, -92.5486) projected
  arc A249 (39.937, -94.1354) -> (40.7196, -92.5486) centre (38.7196, -92.5486) ccw projected
  arc A250 (39.937, -94.1354) -> (39.7673, -94.2779) centre (41.4696, -96.1328) ccw projected
  arc A251 (39.7673, -94.2779) -> (39.1196, -95.7515) centre (41.1196, -95.7515) ccw projected
  line L226 (39.1196, -95.7515) -> (39.1196, -100.7076) projected
  arc A252 (39.1196, -100.7076) -> (39.7673, -102.1811) centre (41.1196, -100.7076) ccw projected
  arc A253 (39.7673, -102.1811) -> (40.773, -102.7455) centre (41.4696, -100.3262) ccw projected
  arc A254 (42.2196, -104.6674) -> (40.773, -102.7455) centre (40.2196, -104.6674) ccw projected
  line L227 (42.2196, -104.6674) -> (42.2196, -114.1237) projected
  arc A255 (42.2196, -114.1237) -> (43.2196, -115.1237) centre (43.2196, -114.1237) ccw projected
  line L228 (43.2196, -115.1237) -> (58.5858, -115.1237) projected
  arc A256 (58.5858, -115.1237) -> (59.2929, -114.8308) centre (58.5858, -114.1237) ccw projected
  line L229 (59.2929, -114.8308) -> (63.7071, -110.4166) projected
  arc A257 (63.7071, -110.4166) -> (64, -109.7094) centre (63, -109.7094) ccw projected
  line L230 (-69.3194, 207.0635) -> (-69.3194, 50.0635) projected
  arc A258 (-69.3194, 50.0635) -> (-68.3194, 49.0635) centre (-68.3194, 50.0635) ccw projected
  line L231 (-68.3194, 49.0635) -> (-25.6194, 49.0635) projected
  arc A259 (-25.6194, 49.0635) -> (-24.6194, 50.0635) centre (-25.6194, 50.0635) ccw projected
  line L232 (-24.6194, 50.0635) -> (-24.6194, 207.0635) projected
  arc A260 (-24.6194, 207.0635) -> (-25.6194, 208.0635) centre (-25.6194, 207.0635) ccw projected
  line L233 (-25.6194, 208.0635) -> (-68.3194, 208.0635) projected
  arc A261 (-68.3194, 208.0635) -> (-69.3194, 207.0635) centre (-68.3194, 207.0635) ccw projected
  arc A262 (31.7396, -114.6081) -> (34.7396, -111.6081) centre (31.7396, -111.6081) ccw projected
  line L234 (34.7396, -111.6081) -> (34.7396, -101.7281) projected
  arc A263 (34.7396, -101.7281) -> (31.7396, -98.7281) centre (31.7396, -101.7281) ccw projected
  line L235 (31.7396, -98.7281) -> (-55.9404, -98.7281) projected
  arc A264 (-55.9404, -98.7281) -> (-58.9404, -101.7281) centre (-55.9404, -101.7281) ccw projected
  line L236 (-58.9404, -101.7281) -> (-58.9404, -111.6081) projected
  arc A265 (-58.9404, -111.6081) -> (-55.9404, -114.6081) centre (-55.9404, -111.6081) ccw projected
  line L237 (-55.9404, -114.6081) -> (31.7396, -114.6081) projected
  arc A266 (34.7396, -81.3827) -> (31.7396, -78.3827) centre (31.7396, -81.3827) ccw projected
  line L238 (31.7396, -78.3827) -> (-55.9404, -78.3827) projected
  arc A267 (-55.9404, -78.3827) -> (-58.9404, -81.3827) centre (-55.9404, -81.3827) ccw projected
  line L239 (-58.9404, -81.3827) -> (-58.9404, -91.2627) projected
  arc A268 (-58.9404, -91.2627) -> (-55.9404, -94.2627) centre (-55.9404, -91.2627) ccw projected
  line L240 (-55.9404, -94.2627) -> (31.7396, -94.2627) projected
  arc A269 (31.7396, -94.2627) -> (34.7396, -91.2627) centre (31.7396, -91.2627) ccw projected
  line L241 (34.7396, -91.2627) -> (34.7396, -81.3827) projected
  line L242 (-55.9404, -33.2265) -> (31.7396, -33.2265) projected
  arc A270 (31.7396, -33.2265) -> (34.7396, -30.2265) centre (31.7396, -30.2265) ccw projected
  line L243 (34.7396, -30.2265) -> (34.7396, -20.3465) projected
  arc A271 (34.7396, -20.3465) -> (31.7396, -17.3465) centre (31.7396, -20.3465) ccw projected
  line L244 (31.7396, -17.3465) -> (-55.9404, -17.3465) projected
  arc A272 (-55.9404, -17.3465) -> (-58.9404, -20.3465) centre (-55.9404, -20.3465) ccw projected
  line L245 (-58.9404, -20.3465) -> (-58.9404, -30.2265) projected
  arc A273 (-58.9404, -30.2265) -> (-55.9404, -33.2265) centre (-55.9404, -30.2265) ccw projected
  line L246 (31.7396, -58.0373) -> (-55.9404, -58.0373) projected
  arc A274 (-55.9404, -58.0373) -> (-58.9404, -61.0373) centre (-55.9404, -61.0373) ccw projected
  line L247 (-58.9404, -61.0373) -> (-58.9404, -70.9173) projected
  arc A275 (-58.9404, -70.9173) -> (-55.9404, -73.9173) centre (-55.9404, -70.9173) ccw projected
  line L248 (-55.9404, -73.9173) -> (31.7396, -73.9173) projected
  arc A276 (31.7396, -73.9173) -> (34.7396, -70.9173) centre (31.7396, -70.9173) ccw projected
  line L249 (34.7396, -70.9173) -> (34.7396, -61.0373) projected
  arc A277 (34.7396, -61.0373) -> (31.7396, -58.0373) centre (31.7396, -61.0373) ccw projected
  arc A278 (-55.9404, -37.6919) -> (-58.9404, -40.6919) centre (-55.9404, -40.6919) ccw projected
  line L250 (-58.9404, -40.6919) -> (-58.9404, -50.5719) projected
  arc A279 (-58.9404, -50.5719) -> (-55.9404, -53.5719) centre (-55.9404, -50.5719) ccw projected
  line L251 (-55.9404, -53.5719) -> (31.7396, -53.5719) projected
  arc A280 (31.7396, -53.5719) -> (34.7396, -50.5719) centre (31.7396, -50.5719) ccw projected
  line L252 (34.7396, -50.5719) -> (34.7396, -40.6919) projected
  arc A281 (34.7396, -40.6919) -> (31.7396, -37.6919) centre (31.7396, -40.6919) ccw projected
  line L253 (31.7396, -37.6919) -> (-55.9404, -37.6919) projected
  arc A282 (-55.9404, 2.9989) -> (-58.9404, -0.0011) centre (-55.9404, -0.0011) ccw projected
  line L254 (-58.9404, -0.0011) -> (-58.9404, -9.8811) projected
  arc A283 (-58.9404, -9.8811) -> (-55.9404, -12.8811) centre (-55.9404, -9.8811) ccw projected
  line L255 (-55.9404, -12.8811) -> (31.7396, -12.8811) projected
  arc A284 (31.7396, -12.8811) -> (34.7396, -9.8811) centre (31.7396, -9.8811) ccw projected
  line L256 (34.7396, -9.8811) -> (34.7396, -0.0011) projected
  arc A285 (34.7396, -0.0011) -> (31.7396, 2.9989) centre (31.7396, -0.0011) ccw projected
  line L257 (31.7396, 2.9989) -> (-55.9404, 2.9989) projected
  line L258 (-58.9404, 40.6897) -> (-58.9404, 30.8097) projected
  arc A286 (-58.9404, 30.8097) -> (-55.9404, 27.8097) centre (-55.9404, 30.8097) ccw projected
  line L259 (-55.9404, 27.8097) -> (31.7396, 27.8097) projected
  arc A287 (31.7396, 27.8097) -> (34.7396, 30.8097) centre (31.7396, 30.8097) ccw projected
  line L260 (34.7396, 30.8097) -> (34.7396, 40.6897) projected
  arc A288 (34.7396, 40.6897) -> (31.7396, 43.6897) centre (31.7396, 40.6897) ccw projected
  line L261 (31.7396, 43.6897) -> (-55.9404, 43.6897) projected
  arc A289 (-55.9404, 43.6897) -> (-58.9404, 40.6897) centre (-55.9404, 40.6897) ccw projected
  line L262 (-58.9404, 20.3443) -> (-58.9404, 10.4643) projected
  arc A290 (-58.9404, 10.4643) -> (-55.9404, 7.4643) centre (-55.9404, 10.4643) ccw projected
  line L263 (-55.9404, 7.4643) -> (31.7396, 7.4643) projected
  arc A291 (31.7396, 7.4643) -> (34.7396, 10.4643) centre (31.7396, 10.4643) ccw projected
  line L264 (34.7396, 10.4643) -> (34.7396, 20.3443) projected
  arc A292 (34.7396, 20.3443) -> (31.7396, 23.3443) centre (31.7396, 20.3443) ccw projected
  line L265 (31.7396, 23.3443) -> (-55.9404, 23.3443) projected
  arc A293 (-55.9404, 23.3443) -> (-58.9404, 20.3443) centre (-55.9404, 20.3443) ccw projected
  circle A294 centre (16.1067, -140) radius 2.25 projected
  circle A295 centre (-17.8933, -140) radius 2.25 projected
  line L266 (-75, 46.0635) -> (-78, 46.0635) projected
  line L267 (-78, 46.0635) -> (-78, 215) projected
  line L268 (-78, 215) -> (80.4, 215) projected
  line L269 (80.4, 215) -> (80.4, 184.5) projected
  line L270 (80.4, 184.5) -> (98, 184.5) projected
  line L271 (98, 184.5) -> (98, -129) projected
  line L272 (98, -129) -> (23.6067, -129) projected
  line L273 (23.6067, -129) -> (23.6067, -146.5) projected
  line L274 (23.6067, -146.5) -> (-25.3933, -146.5) projected
  line L275 (-25.3933, -146.5) -> (-25.3933, -129) projected
  line L276 (-25.3933, -129) -> (-75, -129) projected
  line L277 (-75, -129) -> (-75, -112.7392) projected
  line L278 (-75, -112.7392) -> (-78, -112.7392) projected
  line L279 (-78, -112.7392) -> (-78, -102.4522) projected
  line L280 (-78, -102.4522) -> (-75, -102.4522) projected
  line L281 (-75, -102.4522) -> (-75, -92.3938) projected
  line L282 (-75, -92.3938) -> (-78, -92.3938) projected
  line L283 (-78, -92.3938) -> (-78, -82.1068) projected
  line L284 (-78, -82.1068) -> (-75, -82.1068) projected
  line L285 (-75, -82.1068) -> (-75, -71.7392) projected
  line L286 (-75, -71.7392) -> (-78, -71.7392) projected
  line L287 (-78, -71.7392) -> (-78, -61.4522) projected
  line L288 (-78, -61.4522) -> (-75, -61.4522) projected
  line L289 (-75, -61.4522) -> (-75, -51.3938) projected
  line L290 (-75, -51.3938) -> (-78, -51.3938) projected
  line L291 (-78, -51.3938) -> (-78, -41.1068) projected
  line L292 (-78, -41.1068) -> (-75, -41.1068) projected
  line L293 (-75, -41.1068) -> (-75, -30.7392) projected
  line L294 (-75, -30.7392) -> (-78, -30.7392) projected
  line L295 (-78, -30.7392) -> (-78, -20.4522) projected
  line L296 (-78, -20.4522) -> (-75, -20.4522) projected
  line L297 (-75, -20.4522) -> (-75, -10.3938) projected
  line L298 (-75, -10.3938) -> (-78, -10.3938) projected
  line L299 (-78, -10.3938) -> (-78, -0.1068) projected
  line L300 (-78, -0.1068) -> (-75, -0.1068) projected
  line L301 (-75, -0.1068) -> (-75, 10.2608) projected
  line L302 (-75, 10.2608) -> (-78, 10.2608) projected
  line L303 (-78, 10.2608) -> (-78, 20.5478) projected
  line L304 (-78, 20.5478) -> (-75, 20.5478) projected
  line L305 (-75, 20.5478) -> (-75, 30.6062) projected
  line L306 (-75, 30.6062) -> (-78, 30.6062) projected
  line L307 (-78, 30.6062) -> (-78, 40.8932) projected
  line L308 (-78, 40.8932) -> (-75, 40.8932) projected
  line L309 (-75, 40.8932) -> (-75, 46.0635) projected
  circle A296 centre (88, -117.6237) radius 2.25 projected
  circle A297 centre (88, 58.3987) radius 2.25 projected
  circle A298 centre (88, 131.8987) radius 2.25 projected
  circle A299 centre (88, 174.5) radius 2.25 projected
  line L310 (64, -109.7094) -> (64, 48.3987) projected
  line L311 (64, 48.3987) -> (44.819, 48.3987) projected
  arc A300 (43.3362, 49.0566) -> (44.819, 48.3987) centre (44.819, 50.3987) ccw projected
  arc A301 (43.3362, 49.0566) -> (39.7673, 49.2221) centre (41.4696, 47.3672) ccw projected
  arc A302 (39.7673, 49.2221) -> (39.1196, 47.7485) centre (41.1196, 47.7485) ccw projected
  line L312 (39.1196, 47.7485) -> (39.1196, 42.7924) projected
  arc A303 (39.1196, 42.7924) -> (39.7673, 41.3189) centre (41.1196, 42.7924) ccw projected
  arc A304 (39.7673, 41.3189) -> (39.937, 41.1764) centre (41.4696, 43.1738) ccw projected
  arc A305 (40.7196, 39.5896) -> (39.937, 41.1764) centre (38.7196, 39.5896) ccw projected
  line L313 (40.7196, 39.5896) -> (40.7196, 30.4514) projected
  arc A306 (39.937, 28.8646) -> (40.7196, 30.4514) centre (38.7196, 30.4514) ccw projected
  arc A307 (39.937, 28.8646) -> (39.7673, 28.7221) centre (41.4696, 26.8672) ccw projected
  arc A308 (39.7673, 28.7221) -> (39.1196, 27.2485) centre (41.1196, 27.2485) ccw projected
  line L314 (39.1196, 27.2485) -> (39.1196, 22.2924) projected
  arc A309 (39.1196, 22.2924) -> (39.7673, 20.8189) centre (41.1196, 22.2924) ccw projected
  arc A310 (39.7673, 20.8189) -> (39.937, 20.6764) centre (41.4696, 22.6738) ccw projected
  arc A311 (40.7196, 19.0896) -> (39.937, 20.6764) centre (38.7196, 19.0896) ccw projected
  line L315 (40.7196, 19.0896) -> (40.7196, 9.9514) projected
  arc A312 (39.937, 8.3646) -> (40.7196, 9.9514) centre (38.7196, 9.9514) ccw projected
  arc A313 (39.937, 8.3646) -> (39.7673, 8.2221) centre (41.4696, 6.3672) ccw projected
  arc A314 (39.7673, 8.2221) -> (39.1196, 6.7485) centre (41.1196, 6.7485) ccw projected
  line L316 (39.1196, 6.7485) -> (39.1196, 1.7924) projected
  arc A315 (39.1196, 1.7924) -> (39.7673, 0.3189) centre (41.1196, 1.7924) ccw projected
  arc A316 (39.7673, 0.3189) -> (39.937, 0.1764) centre (41.4696, 2.1738) ccw projected
  arc A317 (40.7196, -1.4104) -> (39.937, 0.1764) centre (38.7196, -1.4104) ccw projected
  line L317 (40.7196, -1.4104) -> (40.7196, -10.5486) projected
  arc A318 (39.937, -12.1354) -> (40.7196, -10.5486) centre (38.7196, -10.5486) ccw projected
  arc A319 (39.937, -12.1354) -> (39.7673, -12.2779) centre (41.4696, -14.1328) ccw projected
  arc A320 (39.7673, -12.2779) -> (39.1196, -13.7515) centre (41.1196, -13.7515) ccw projected
  line L318 (39.1196, -13.7515) -> (39.1196, -18.7076) projected
  arc A321 (39.1196, -18.7076) -> (39.7673, -20.1811) centre (41.1196, -18.7076) ccw projected
  arc A322 (39.7673, -20.1811) -> (39.937, -20.3236) centre (41.4696, -18.3262) ccw projected
  arc A323 (40.7196, -21.9104) -> (39.937, -20.3236) centre (38.7196, -21.9104) ccw projected
  line L319 (40.7196, -21.9104) -> (40.7196, -31.0486) projected
  arc A324 (39.937, -32.6354) -> (40.7196, -31.0486) centre (38.7196, -31.0486) ccw projected
  arc A325 (39.937, -32.6354) -> (39.7673, -32.7779) centre (41.4696, -34.6328) ccw projected
  arc A326 (39.7673, -32.7779) -> (39.1196, -34.2515) centre (41.1196, -34.2515) ccw projected
  line L320 (39.1196, -34.2515) -> (39.1196, -39.2076) projected
  arc A327 (39.1196, -39.2076) -> (39.7673, -40.6811) centre (41.1196, -39.2076) ccw projected
  arc A328 (39.7673, -40.6811) -> (39.937, -40.8236) centre (41.4696, -38.8262) ccw projected
  arc A329 (40.7196, -42.4104) -> (39.937, -40.8236) centre (38.7196, -42.4104) ccw projected
  line L321 (40.7196, -42.4104) -> (40.7196, -51.5486) projected
  arc A330 (39.937, -53.1354) -> (40.7196, -51.5486) centre (38.7196, -51.5486) ccw projected
  arc A331 (39.937, -53.1354) -> (39.7673, -53.2779) centre (41.4696, -55.1328) ccw projected
  arc A332 (39.7673, -53.2779) -> (39.1196, -54.7515) centre (41.1196, -54.7515) ccw projected
  line L322 (39.1196, -54.7515) -> (39.1196, -59.7076) projected
  arc A333 (39.1196, -59.7076) -> (39.7673, -61.1811) centre (41.1196, -59.7076) ccw projected
  arc A334 (39.7673, -61.1811) -> (39.937, -61.3236) centre (41.4696, -59.3262) ccw projected
  arc A335 (40.7196, -62.9104) -> (39.937, -61.3236) centre (38.7196, -62.9104) ccw projected
  line L323 (40.7196, -62.9104) -> (40.7196, -72.0486) projected
  arc A336 (39.937, -73.6354) -> (40.7196, -72.0486) centre (38.7196, -72.0486) ccw projected
  arc A337 (39.937, -73.6354) -> (39.7673, -73.7779) centre (41.4696, -75.6328) ccw projected
  arc A338 (39.7673, -73.7779) -> (39.1196, -75.2515) centre (41.1196, -75.2515) ccw projected
  line L324 (39.1196, -75.2515) -> (39.1196, -80.2076) projected
  arc A339 (39.1196, -80.2076) -> (39.7673, -81.6811) centre (41.1196, -80.2076) ccw projected
  arc A340 (39.7673, -81.6811) -> (39.937, -81.8236) centre (41.4696, -79.8262) ccw projected
  arc A341 (40.7196, -83.4104) -> (39.937, -81.8236) centre (38.7196, -83.4104) ccw projected
  line L325 (40.7196, -83.4104) -> (40.7196, -92.5486) projected
  arc A342 (39.937, -94.1354) -> (40.7196, -92.5486) centre (38.7196, -92.5486) ccw projected
  arc A343 (39.937, -94.1354) -> (39.7673, -94.2779) centre (41.4696, -96.1328) ccw projected
  arc A344 (39.7673, -94.2779) -> (39.1196, -95.7515) centre (41.1196, -95.7515) ccw projected
  line L326 (39.1196, -95.7515) -> (39.1196, -100.7076) projected
  arc A345 (39.1196, -100.7076) -> (39.7673, -102.1811) centre (41.1196, -100.7076) ccw projected
  arc A346 (39.7673, -102.1811) -> (40.773, -102.7455) centre (41.4696, -100.3262) ccw projected
  arc A347 (42.2196, -104.6674) -> (40.773, -102.7455) centre (40.2196, -104.6674) ccw projected
  line L327 (42.2196, -104.6674) -> (42.2196, -114.1237) projected
  arc A348 (42.2196, -114.1237) -> (43.2196, -115.1237) centre (43.2196, -114.1237) ccw projected
  line L328 (43.2196, -115.1237) -> (58.5858, -115.1237) projected
  arc A349 (58.5858, -115.1237) -> (59.2929, -114.8308) centre (58.5858, -114.1237) ccw projected
  line L329 (59.2929, -114.8308) -> (63.7071, -110.4166) projected
  arc A350 (63.7071, -110.4166) -> (64, -109.7094) centre (63, -109.7094) ccw projected
  line L330 (-69.3194, 207.0635) -> (-69.3194, 50.0635) projected
  arc A351 (-69.3194, 50.0635) -> (-68.3194, 49.0635) centre (-68.3194, 50.0635) ccw projected
  line L331 (-68.3194, 49.0635) -> (-25.6194, 49.0635) projected
  arc A352 (-25.6194, 49.0635) -> (-24.6194, 50.0635) centre (-25.6194, 50.0635) ccw projected
  line L332 (-24.6194, 50.0635) -> (-24.6194, 207.0635) projected
  arc A353 (-24.6194, 207.0635) -> (-25.6194, 208.0635) centre (-25.6194, 207.0635) ccw projected
  line L333 (-25.6194, 208.0635) -> (-68.3194, 208.0635) projected
  arc A354 (-68.3194, 208.0635) -> (-69.3194, 207.0635) centre (-68.3194, 207.0635) ccw projected
  arc A355 (31.7396, -114.6081) -> (34.7396, -111.6081) centre (31.7396, -111.6081) ccw projected
  line L334 (34.7396, -111.6081) -> (34.7396, -101.7281) projected
  arc A356 (34.7396, -101.7281) -> (31.7396, -98.7281) centre (31.7396, -101.7281) ccw projected
  line L335 (31.7396, -98.7281) -> (-55.9404, -98.7281) projected
  arc A357 (-55.9404, -98.7281) -> (-58.9404, -101.7281) centre (-55.9404, -101.7281) ccw projected
  line L336 (-58.9404, -101.7281) -> (-58.9404, -111.6081) projected
  arc A358 (-58.9404, -111.6081) -> (-55.9404, -114.6081) centre (-55.9404, -111.6081) ccw projected
  line L337 (-55.9404, -114.6081) -> (31.7396, -114.6081) projected
  arc A359 (34.7396, -81.3827) -> (31.7396, -78.3827) centre (31.7396, -81.3827) ccw projected
  line L338 (31.7396, -78.3827) -> (-55.9404, -78.3827) projected
  arc A360 (-55.9404, -78.3827) -> (-58.9404, -81.3827) centre (-55.9404, -81.3827) ccw projected
  line L339 (-58.9404, -81.3827) -> (-58.9404, -91.2627) projected
  arc A361 (-58.9404, -91.2627) -> (-55.9404, -94.2627) centre (-55.9404, -91.2627) ccw projected
  line L340 (-55.9404, -94.2627) -> (31.7396, -94.2627) projected
  arc A362 (31.7396, -94.2627) -> (34.7396, -91.2627) centre (31.7396, -91.2627) ccw projected
  line L341 (34.7396, -91.2627) -> (34.7396, -81.3827) projected
  line L342 (-55.9404, -33.2265) -> (31.7396, -33.2265) projected
  arc A363 (31.7396, -33.2265) -> (34.7396, -30.2265) centre (31.7396, -30.2265) ccw projected
  line L343 (34.7396, -30.2265) -> (34.7396, -20.3465) projected
  arc A364 (34.7396, -20.3465) -> (31.7396, -17.3465) centre (31.7396, -20.3465) ccw projected
  line L344 (31.7396, -17.3465) -> (-55.9404, -17.3465) projected
  arc A365 (-55.9404, -17.3465) -> (-58.9404, -20.3465) centre (-55.9404, -20.3465) ccw projected
  line L345 (-58.9404, -20.3465) -> (-58.9404, -30.2265) projected
  arc A366 (-58.9404, -30.2265) -> (-55.9404, -33.2265) centre (-55.9404, -30.2265) ccw projected
  line L346 (31.7396, -58.0373) -> (-55.9404, -58.0373) projected
  arc A367 (-55.9404, -58.0373) -> (-58.9404, -61.0373) centre (-55.9404, -61.0373) ccw projected
  line L347 (-58.9404, -61.0373) -> (-58.9404, -70.9173) projected
  arc A368 (-58.9404, -70.9173) -> (-55.9404, -73.9173) centre (-55.9404, -70.9173) ccw projected
  line L348 (-55.9404, -73.9173) -> (31.7396, -73.9173) projected
  arc A369 (31.7396, -73.9173) -> (34.7396, -70.9173) centre (31.7396, -70.9173) ccw projected
  line L349 (34.7396, -70.9173) -> (34.7396, -61.0373) projected
  arc A370 (34.7396, -61.0373) -> (31.7396, -58.0373) centre (31.7396, -61.0373) ccw projected
  arc A371 (-55.9404, -37.6919) -> (-58.9404, -40.6919) centre (-55.9404, -40.6919) ccw projected
  line L350 (-58.9404, -40.6919) -> (-58.9404, -50.5719) projected
  arc A372 (-58.9404, -50.5719) -> (-55.9404, -53.5719) centre (-55.9404, -50.5719) ccw projected
  line L351 (-55.9404, -53.5719) -> (31.7396, -53.5719) projected
  arc A373 (31.7396, -53.5719) -> (34.7396, -50.5719) centre (31.7396, -50.5719) ccw projected
  line L352 (34.7396, -50.5719) -> (34.7396, -40.6919) projected
  arc A374 (34.7396, -40.6919) -> (31.7396, -37.6919) centre (31.7396, -40.6919) ccw projected
  line L353 (31.7396, -37.6919) -> (-55.9404, -37.6919) projected
  arc A375 (-55.9404, 2.9989) -> (-58.9404, -0.0011) centre (-55.9404, -0.0011) ccw projected
  line L354 (-58.9404, -0.0011) -> (-58.9404, -9.8811) projected
  arc A376 (-58.9404, -9.8811) -> (-55.9404, -12.8811) centre (-55.9404, -9.8811) ccw projected
  line L355 (-55.9404, -12.8811) -> (31.7396, -12.8811) projected
  arc A377 (31.7396, -12.8811) -> (34.7396, -9.8811) centre (31.7396, -9.8811) ccw projected
  line L356 (34.7396, -9.8811) -> (34.7396, -0.0011) projected
  arc A378 (34.7396, -0.0011) -> (31.7396, 2.9989) centre (31.7396, -0.0011) ccw projected
  line L357 (31.7396, 2.9989) -> (-55.9404, 2.9989) projected
  line L358 (-58.9404, 40.6897) -> (-58.9404, 30.8097) projected
  arc A379 (-58.9404, 30.8097) -> (-55.9404, 27.8097) centre (-55.9404, 30.8097) ccw projected
  line L359 (-55.9404, 27.8097) -> (31.7396, 27.8097) projected
  arc A380 (31.7396, 27.8097) -> (34.7396, 30.8097) centre (31.7396, 30.8097) ccw projected
  line L360 (34.7396, 30.8097) -> (34.7396, 40.6897) projected
  arc A381 (34.7396, 40.6897) -> (31.7396, 43.6897) centre (31.7396, 40.6897) ccw projected
  line L361 (31.7396, 43.6897) -> (-55.9404, 43.6897) projected
  arc A382 (-55.9404, 43.6897) -> (-58.9404, 40.6897) centre (-55.9404, 40.6897) ccw projected
  line L362 (-58.9404, 20.3443) -> (-58.9404, 10.4643) projected
  arc A383 (-58.9404, 10.4643) -> (-55.9404, 7.4643) centre (-55.9404, 10.4643) ccw projected